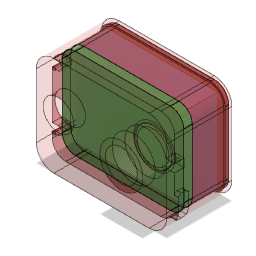
MDCEnclosure (Autodesk Fusion 360 design; units mm, degrees)
Autodesk Fusion 360 part; units mm, degrees
sketch "Board" plane through (0, 0, 0) normal (0, 0, 1) x (1, 0, 0)
  line L0 (4.75, 0) -> (39.105, 0)
  line L1 (43.855, 4.75) -> (43.855, 27.9)
  line L2 (39.105, 32.65) -> (4.75, 32.65)
  line L3 (0, 27.9) -> (0, 4.75)
  arc A0 (4.75, 32.65) -> (0, 27.9) centre (4.75, 27.9) ccw
  arc A1 (43.855, 27.9) -> (39.105, 32.65) centre (39.105, 27.9) ccw
  arc A2 (39.105, 0) -> (43.855, 4.75) centre (39.105, 4.75) ccw
  arc A3 (0, 4.75) -> (4.75, 0) centre (4.75, 4.75) ccw
  line L4 (-0.15, 27.9) -> (-0.15, 4.75)
  arc A4 (-0.15, 4.75) -> (4.75, -0.15) centre (4.75, 4.75) ccw
  line L5 (4.75, -0.15) -> (39.105, -0.15)
  arc A5 (39.105, -0.15) -> (44.005, 4.75) centre (39.105, 4.75) ccw
  line L6 (44.005, 4.75) -> (44.005, 27.9)
  arc A6 (44.005, 27.9) -> (39.105, 32.8) centre (39.105, 27.9) ccw
  line L7 (39.105, 32.8) -> (4.75, 32.8)
  arc A7 (4.75, 32.8) -> (-0.15, 27.9) centre (4.75, 27.9) ccw
  line L8 (-0.35, 27.9) -> (-0.35, 4.75)
  arc A8 (-0.35, 4.75) -> (4.75, -0.35) centre (4.75, 4.75) ccw
  line L9 (4.75, -0.35) -> (39.105, -0.35)
  arc A9 (39.105, -0.35) -> (44.205, 4.75) centre (39.105, 4.75) ccw
  line L10 (44.205, 4.75) -> (44.205, 27.9)
  arc A10 (44.205, 27.9) -> (39.105, 33) centre (39.105, 27.9) ccw
  line L11 (39.105, 33) -> (4.75, 33)
  arc A11 (4.75, 33) -> (-0.35, 27.9) centre (4.75, 27.9) ccw
  line L12 (-0.5, 27.9) -> (-0.5, 4.75)
  arc A12 (-0.5, 4.75) -> (4.75, -0.5) centre (4.75, 4.75) ccw
  line L13 (4.75, -0.5) -> (39.105, -0.5)
  arc A13 (39.105, -0.5) -> (44.355, 4.75) centre (39.105, 4.75) ccw
  line L14 (44.355, 4.75) -> (44.355, 27.9)
  arc A14 (44.355, 27.9) -> (39.105, 33.15) centre (39.105, 27.9) ccw
  line L15 (39.105, 33.15) -> (4.75, 33.15)
  arc A15 (4.75, 33.15) -> (-0.5, 27.9) centre (4.75, 27.9) ccw
  line L16 (21.9275, 32.65) -> (21.9275, 0)
  point P0 (21.9275, 16.325)
  dimension "d329" = 43.855
  dimension "d330" = 32.65
  dimension "d331" = 4.75
  dimension "d332" = 0.15
  dimension "d336" = 0.35
  dimension "d337" = 0.5
  constraint horizontal L0
  constraint vertical L1
  constraint horizontal L2
  constraint vertical L3
  constraint tangent L2 A0
  constraint tangent L3 A0
  constraint tangent L1 A1
  constraint tangent L2 A1
  constraint equal A0 A1
  constraint tangent L0 A2
  constraint tangent L1 A2
  constraint equal A0 A2
  constraint tangent L0 A3
  constraint tangent L3 A3
  constraint equal A0 A3
  constraint midpoint L2 L16.start
  constraint midpoint L0 L16.end
  constraint midpoint L16 P0
  measures "d329" distance of L1 L3
  measures "d330" distance of L0 L2
  measures "d331" radius of A0
ref_plane "WorkPlane7" through (21.9275, 16.325, -3.46) normal (0, 0, 1) x (1, 0, 0)
sketch "MountPoints" plane through (0, 0, -3.46) normal (0, 0, 1) x (1, 0, 0)
  line L0 (-0.15, 29.9) -> (0.44, 29.9)
  line L1 (0.44, 29.9) -> (0.44, 26.9)
  line L2 (0.44, 26.9) -> (-0.15, 26.9)
  line L3 (-0.15, 26.9) -> (-0.15, 29.9)
  line L4 (0.44, 29.9) -> (1.94, 29.9)
  line L5 (3.44, 28.4) -> (3.44, 28.4)
  line L6 (1.94, 26.9) -> (0.44, 26.9)
  line L7 (0.44, 26.9) -> (0.44, 29.9)
  line L8 (0.39, 9.672) -> (1.89, 9.672)
  line L9 (3.39, 8.172) -> (3.39, 8.172)
  line L10 (1.89, 6.672) -> (0.39, 6.672)
  line L11 (0.39, 6.672) -> (0.39, 9.672)
  line L12 (-0.15, 9.672) -> (0.39, 9.672)
  line L13 (0.39, 9.672) -> (0.39, 6.672)
  line L14 (0.39, 6.672) -> (-0.15, 6.672)
  line L15 (-0.15, 6.672) -> (-0.15, 9.672)
  line L16 (-0.15, 27.9) -> (-0.15, 4.75)
  line L17 (44.005, 4.75) -> (44.005, 27.9)
  line L18 (4.75, -0.15) -> (39.105, -0.15)
  line L19 (0.44, 28.4) -> (3.44, 28.4) construction
  line L20 (0.39, 8.172) -> (3.39, 8.172) construction
  line L21 (0, 27.9) -> (0, 4.75) construction
  line L22 (4.75, 0) -> (39.105, 0) construction
  arc A0 (3.44, 28.4) -> (1.94, 29.9) centre (1.94, 28.4) ccw
  arc A1 (1.94, 26.9) -> (3.44, 28.4) centre (1.94, 28.4) ccw
  arc A2 (3.39, 8.172) -> (1.89, 9.672) centre (1.89, 8.172) ccw
  arc A3 (1.89, 6.672) -> (3.39, 8.172) centre (1.89, 8.172) ccw
  line L23 (44.005, 18.892) -> (38.505, 18.892)
  line L24 (38.505, 18.892) -> (38.505, 15.892)
  line L25 (38.505, 15.892) -> (44.005, 15.892)
  line L26 (44.005, 15.892) -> (44.005, 18.892)
  line L27 (44.005, 4.75) -> (44.005, 27.9)
  line L28 (4.75, 0) -> (39.105, 0)
  line L29 (0, 27.9) -> (0, 4.75)
  line L30 (44.005, 17.392) -> (38.505, 17.392)
  point P0 (1.94, 28.4)
  point P1 (1.89, 8.172)
  point P2 (41.9, 17.392)
  dimension "d404" = 3
  dimension "d411" = 3
  dimension "d412" = 1.89
  dimension "d413" = 8.172
  dimension "d418" = 1.94
  dimension "d419" = 28.4
  dimension "d422" = 1.5
  dimension "d572" = 5.5
  dimension "d608" = 17.392
  dimension "d609" = 41.9
  dimension "d610" = 3
  constraint horizontal L0
  constraint vertical L1
  constraint horizontal L2
  constraint vertical L3
  constraint horizontal L4
  constraint horizontal L6
  constraint vertical L7
  constraint horizontal L8
  constraint horizontal L10
  constraint vertical L11
  constraint horizontal L12
  constraint vertical L13
  constraint horizontal L14
  constraint vertical L15
  constraint collinear L1 L7
  constraint collinear L0 L4
  constraint collinear L2 L6
  constraint collinear L3 L16
  constraint collinear L11 L13
  constraint collinear L8 L12
  constraint collinear L10 L14
  constraint collinear L15 L16
  constraint midpoint L1 L19.start
  constraint midpoint L13 L20.start
  constraint midpoint L19 P0
  constraint midpoint L20 P1
  constraint tangent L4 A0
  constraint tangent L6 A1
  constraint equal A0 A1
  constraint tangent L8 A2
  constraint equal A0 A2
  constraint tangent L10 A3
  constraint equal A0 A3
  constraint horizontal L23
  constraint vertical L24
  constraint horizontal L25
  constraint vertical L26
  constraint midpoint L26 L30.start
  constraint midpoint L24 L30.end
  constraint coincident P2 L30
  constraint collinear L26 L27
  measures "d404" distance of L4 L6
  measures "d411" distance of L8 L10
  measures "d412" distance of P1 L21
  measures "d413" distance of P1 L22
  measures "d418" distance of P0 L21
  measures "d419" distance of P0 L22
  measures "d422" radius of A0
  measures "d572" distance of L24 L26
  measures "d608" distance of P2 L28
  measures "d609" distance of P2 L29
  measures "d610" distance of L23 L25
extrude "Front-Sidewalls" add sketch "Board" along normal blind 23.56 thin wall 1.5 on the left open curves L4 A4 L5 A5 L6 A6 L7 A7 makes body 1 in component "Front"
sketch "FrontHoles" plane through (0, 0, 0) normal (0, 0, 1) x (1, 0, 0)
  line L0 (0, 27.9) -> (0, 4.75)
  line L1 (4.75, 0) -> (39.105, 0)
  circle A0 centre (33.5424, 17.392) radius 7.5144
  circle A1 centre (33.5424, 17.392) radius 7.7644
  circle A2 centre (33.5424, 17.392) radius 6.75
  point P0 (6.2926, 17.392)
  point P1 (33.5424, 17.392)
  dimension "d350" = 6.2926
  dimension "d351" = 17.392
  dimension "d352" = 33.5424
  dimension "d353" = 17.392
  dimension "d554" = 15.0287
  dimension "d555" = 15.5287
  dimension "d575" = 13.5
  constraint coincident P1 A0.centre
  measures "d350" distance of P0 L0
  measures "d351" distance of P0 L1
  measures "d352" distance of P1 L0
  measures "d353" distance of P1 L1
  measures "d554" diameter of A0
  measures "d555" diameter of A1
  measures "d575" diameter of A2
extrude "Front-Frontplate" add sketch "Board" along normal blind 4.3 separate body contours L0 L2 L3 A0 A3 L16 | L0 L1 L2 A1 A2 L16 | L4 A4 L5 A5 L6 A6 L7 A7 makes body 2 in component "Front"
hole "Front-MotionSensorHole" at (6.2926, 17.392, 0) direction (0, 0, 1) diameter 11 depth 12 tip angle 118 bodies 2 in component "Front"
extrude "Front-LensProtrusionInside" [suppressed]
extrude "Extrude12" add sketch "FrontHoles" against normal blind 3.46 contours A0 | A2 bodies 2 in component "Front"
extrude "Front-BoardMountPoints" [suppressed]
extrude "Extrude16" add sketch "MountPoints" along normal blind 3.46 contours L0 L1 L2 L3 L7 L16 | L1 L4 L6 L7 A0 A1 | L12 L14 L15 L16 L29 | L11 L12 L13 L14 L29 | L8 L10 L11 L13 A2 A3 | L17 L24 L25 L26 L27 L30 | L17 L23 L24 L26 L27 L30 bodies 2 in component "Front"
extrude "Front-LensProtrusionBoardGap" cut sketch "FrontHoles" along normal blind 0.25 from surface at -3.46 contours A0 | A2 bodies 2 in component "Front"
extrude "Extrude24" [no effect]
extrude "Extrude18" cut sketch "FrontHoles" along normal blind 0.5 from surface at -3.21 contours A2 bodies 2 1 in component "Front"
extrude "Front-LensProtrusionOutside" [suppressed]
extrude "Extrude13" add sketch "FrontHoles" along normal blind 8.74 contours A0 | A1 | A2 bodies 2 in component "Front"
hole "Hole8" at (33.5424, 17.392, -3.46) direction (0, 0, 1) diameter 11.529 depth 20 tip angle 180 bodies 2 in component "Front"
thread "Thread2" "ISO Metric profile 12.0 M12x0.5 6H" major diameter 12.0961 minor diameter 11.5287 pitch 0.5 angle 60 resizes the face on face at (33.8297, 23.1493, 1.1067) from (33.5424, 17.392, -0.71) to (33.5424, 17.392, 8.74) on bodies 2 in component "Front"
hole "Hole10" at (1.94, 28.4, -3.46) at (41.9, 17.392, -3.46) at (1.89, 8.172, -3.46) direction (0, 0, 1) diameter 1.271 depth 5 tip angle 180 bodies 2 1 in component "Front"
thread "Thread4" "ISO Metric profile 1.6 M1.6x0.35 6H" major diameter 1.668 minor diameter 1.271 pitch 0.35 angle 60 resizes the face on face at (41.8683, 18.0267, -0.1267) on face at (1.3283, 28.5721, -1.7933) on face at (1.9217, 8.8067, -1.7933) on bodies 2 in component "Front"
move_body "Align7" bodies 2 to x (1, 0, 0) y (0, 1, 0) z (0, 0, 1) at (0, 0, 19.26) in component "Front"
extrude "Front-BackplateInset" cut sketch "Board" along normal blind 1.5 draft 10 contours L0 L2 L3 A0 A3 L16 | L0 L1 L2 A1 A2 L16 | L4 A4 L5 A5 L6 A6 L7 A7 | L8 A8 L9 A9 L10 A10 L11 A11 | L12 A12 L13 A13 L14 A14 L15 A15 bodies 1 in component "Front"
combine "Front-Combine" operation add target body 1 tool bodies 2 in component "Front"
sketch "USBCPlugCutout" plane through (0, 0, 0) normal (1, 0, 0) x (0, 0, -1) in component "Front"
  line L0 (-22, 4.75) -> (-22, 27.9)
  line L1 (-22, 27.9) -> (-23.5, 27.9)
  line L2 (-23.5, 27.9) -> (-23.5, 4.75)
  line L3 (-23.5, 4.75) -> (-22, 4.75)
  line L4 (-18.715, 19.0109) -> (-17.155, 19.0109)
  line L5 (-16.155, 18.0109) -> (-16.155, 10.6709)
  line L6 (-17.155, 9.6709) -> (-18.715, 9.6709)
  line L7 (-19.715, 10.6709) -> (-19.715, 18.0109)
  arc A0 (-18.715, 19.0109) -> (-19.715, 18.0109) centre (-18.715, 18.0109) ccw
  arc A1 (-16.155, 18.0109) -> (-17.155, 19.0109) centre (-17.155, 18.0109) ccw
  arc A2 (-17.155, 9.6709) -> (-16.155, 10.6709) centre (-17.155, 10.6709) ccw
  arc A3 (-19.715, 10.6709) -> (-18.715, 9.6709) centre (-18.715, 10.6709) ccw
  dimension "d492" = 3.56
  dimension "d493" = 9.34
  dimension "d497" = 1
  dimension "d498" = 1
  dimension "d499" = 1
  constraint horizontal L4
  constraint vertical L5
  constraint vertical L7
  constraint tangent L4 A0
  constraint tangent L7 A0
  constraint tangent L4 A1
  constraint tangent L5 A1
  constraint tangent L5 A2
  constraint tangent L6 A2
  constraint tangent L6 A3
  constraint tangent L7 A3
  constraint equal A2 A3
  measures "d492" distance of L5 L7
  measures "d493" distance of L4 L6
  measures "d497" radius of A0
  measures "d498" radius of A1
  measures "d499" radius of A2
extrude "Extrude9" add sketch "USBCPlugCutout" along normal blind 10 separate body contours L4 L5 L6 L7 A0 A1 A2 A3 makes body 3 in component "Front"
ref_plane "WorkPlane5" through (42.4553, 17.392, 15.7) normal (0, 0, -1) x (-1, 0, 0) in component "Front"
ref_plane "WorkPlane6" through (42.005, 16.325, 11.78) normal (-1, 0, 0) x (0, -1, 0) in component "Front"
move_body "Align3" bodies 3 to x (1, 0, 0) y (0, 1, 0) z (0, 0, 1) at (42.005, 0, 0) in component "Front"
move_body "Align4" bodies 3 to x (1, 0, 0) y (0, 1, 0) z (0, 0, 1) at (0, 0, -0.455) in component "Front"
ref_plane "WorkPlane7" through (21.9275, 0, 0) normal (0, -1, 0) x (1, 0, 0) in component "Front"
ref_plane "WorkPlane9" through (21.9275, 5.2535, 0) normal (0, -1, 0) x (1, 0, 0) in component "Front"
move_body "Align5" bodies 3 to x (1, 0, 0) y (0, 1, 0) z (0, 0, 1) at (0, -9.0874, 0) in component "Front"
combine "Combine3" operation cut target body 1 tool bodies 3 in component "Front"
extrude "Back-Backplate" add sketch "Board" along normal blind 1.5 draft 10 separate body contours L0 L2 L3 A0 A3 L16 | L0 L1 L2 A1 A2 L16 | L4 A4 L5 A5 L6 A6 L7 A7 | L8 A8 L9 A9 L10 A10 L11 A11 makes body 4 in component "Back"
sketch "Sketch1" plane through (0, 0, 0) normal (0, 0, 1) x (1, 0, 0) in component "Battery"
  line L0 (20, 15) -> (-20, 15)
  line L1 (-20, 15) -> (-20, -15)
  line L2 (-20, -15) -> (20, -15)
  line L3 (20, -15) -> (20, 15)
  line L4 (20, 15) -> (-20, -15) construction
  dimension "d443" = 40
  dimension "d444" = 30
  constraint horizontal L0
  constraint vertical L1
  constraint horizontal L2
  constraint vertical L3
  constraint midpoint L4 origin
  measures "d443" distance of L1 L3
  measures "d444" distance of L0 L2
extrude "Extrude1" add sketch "Sketch1" along normal blind 11.2 separate body makes body 5 in component "Battery"
move_body "Align1" bodies 5 to x (1, 0, 0) y (0, 1, 0) z (0, 0, 1) at (21.9275, 16.325, 1.5) in component "Battery"
extrude "Extrude1'" add sketch "Board" along normal blind 3.1 separate body contours L0 L2 L3 A0 A3 L16 | L0 L1 L2 A1 A2 L16 makes body 6 in component "Board"
move_body "Align1'" bodies 6 to x (1, 0, 0) y (0, 1, 0) z (0, 0, 1) at (0, 0, 12.7) in component "Board"
component "Front" placed x (1, 0, 0) y (0, 1, 0) z (0, 0, 1) at (0, 0, 0)
component "Back" placed x (1, 0, 0) y (0, 1, 0) z (0, 0, 1) at (0, 0, 0)
component "Battery" placed x (1, 0, 0) y (0, 1, 0) z (0, 0, 1) at (0, 0, 0)
component "Board" placed x (1, 0, 0) y (0, 1, 0) z (0, 0, 1) at (0, 0, 0)
equation "BoardHeight = 32.65 mm"
equation "BoardWidth = 43.855 mm"
equation "EnclosureThickness = 1.5 mm"
equation "ImageSensorX = 33.5424 mm"
equation "ImageSensorY = 17.392 mm"
equation "MotionSensorX = 6.2926 mm"
equation "MotionSensorY = 17.392 mm"
equation "LensHoleDiameter = 15.1 mm + 0.2 mm + EnclosureMfgTol"
equation "MotionSensorDiameter = 10.4 mm + 0.5 mm + EnclosureMfgTol"
equation "LensProtrusionOutsideThickness = 13.5287 mm + 2 mm"
equation "LensProtrusionDepth = LensThreadDepth - MountPointDepth"
equation "OuterEdgeRadius = 6 mm"
equation "BoardRadius = 4.75 mm"
equation "MountPoint2X = 1.89 mm"
equation "MountPoint2Y = 8.172 mm"
equation "MountPointDepth = USBCReceptacleWidth + 0.3 mm"
equation "MountPoint3X = 41.9 mm"
equation "MountPoint3Y = 17.392 mm"
equation "MountPoint1X = 1.94 mm"
equation "MountPoint1Y = 28.4 mm"
equation "BackplateMountPointDepth = EnclosureDepth - FrontplateThickness"
equation "BackplateMountPointWidth = 1.5 mm"
equation "BackplateMountPointChamfer = BackplateMountPointWidth"
equation "HoleDiameter = 1.3 mm"
equation "BatteryWidth = 40 mm"
equation "BatteryHeight = 30 mm"
equation "BatteryThickness = 11 mm + 0.2 mm"
equation "BackplateOverlap = 0.2 mm"
equation "BackplateHoleOffset = 0.1 mm"
equation "ScrewHeadDiameter = 3 mm"
equation "ScrewHeadHeight = 1 mm"
equation "BackplateThickness = 1.5 mm"
equation "EnclosureDepth = FrontplateThickness + MountPointDepth + BoardThickness + BatteryThickness + BackplateThickness"
equation "BoardThickness = 3.1 mm"
equation "BoardEnclosureGap = 0.15 mm"
equation "USBCReceptacleCutoutWidth = USBCReceptacleWidth + USBCReceptacleTolerance + 2 * EnclosureMfgTol"
equation "USBCReceptacleCutoutHeight = USBCReceptacleHeight + USBCReceptacleTolerance + 2 * EnclosureMfgTol"
equation "USBCReceptacleCutoutRadius = 2.4 mm / 2 - 0.2 mm"
equation "USBCReceptacleY = 5.25348125 mm"
equation "USBCReceptacleWidth = 3.16 mm"
equation "d329 = BoardWidth"
equation "d330 = BoardHeight"
equation "d331 = BoardRadius"
equation "d332 = BoardEnclosureGap"
equation "d333 = EnclosureThickness"
equation "d334 = EnclosureDepth"
equation "d336 = BoardEnclosureGap + BackplateOverlap"
equation "d337 = BoardEnclosureGap + BackplateOverlap + 0.15 mm"
equation "d350 = MotionSensorX"
equation "d351 = MotionSensorY"
equation "d352 = ImageSensorX"
equation "d353 = ImageSensorY"
equation "d354 = FrontplateThickness"
equation "d363 = MotionSensorDiameter"
equation "d372 = EnclosureThickness"
equation "MountPointWidth = 3 mm"
equation "MountPointHeight = 3 mm"
equation "MountPointRadius = 1.5 mm"
equation "d404 = MountPointHeight"
equation "d411 = MountPointHeight"
equation "d412 = MountPoint2X"
equation "d413 = MountPoint2Y"
equation "d418 = MountPoint1X"
equation "d419 = MountPoint1Y"
equation "d422 = MountPointRadius"
equation "d426 = BackplateThickness"
equation "d427 = DovetailAngle"
equation "d443 = BatteryWidth"
equation "d444 = BatteryHeight"
equation "d445 = BatteryThickness"
equation "d479 = BoardThickness"
equation "d492 = USBCReceptacleCutoutWidth"
equation "d493 = USBCReceptacleCutoutHeight"
equation "d497 = USBCReceptacleCutoutRadius"
equation "d498 = USBCReceptacleCutoutRadius"
equation "d499 = USBCReceptacleCutoutRadius"
equation "d502 = EnclosureMfgTol"
equation "d505 = -USBCReceptacleY"
equation "USBCReceptacleHeight = 8.94 mm"
equation "USBCReceptacleTolerance = 0.2 mm"
equation "EnclosureMfgTol = 0.1 mm"
equation "FrontplateThickness = 4.3 mm"
equation "LensThreadDepth = 12.2 mm" comment "Lens threaded region length + lens back focal length (BFL)"
equation "LensProtrusionInsideThickness = 13.0287 mm + 2 mm"
equation "d540 = -MountPointDepth"
equation "d542 = -MountPointDepth"
equation "d544 = LensProtrusionDepth"
equation "d546 = LensProtrusionDepth"
equation "d554 = LensProtrusionInsideThickness"
equation "d555 = LensProtrusionOutsideThickness"
equation "BackplateDovetailAngle = 10 deg"
equation "d575 = LensOringOutsideDiameter"
equation "LensOringOutsideDiameter = 13.5 mm"
equation "LensOringThickness = 1 mm"
equation "LensOringSeatDepth = 0.5 mm"
equation "d590 = MountPointDepth"
equation "d592 = MountPointDepth"
equation "d594 = LensProtrusionBoardGap"
equation "d596 = -MountPointDepth"
equation "LensProtrusionBoardGap = 0.25 mm" comment "Gap between inside lens protrusion and board"
equation "d598 = -MountPointDepth + LensProtrusionBoardGap"
equation "d599 = LensOringSeatDepth"
equation "d601 = -MountPointDepth"
equation "d602 = LensProtrusionBoardGap"
equation "d604 = MountPointHoleDepth"
equation "d608 = MountPoint3Y"
equation "d609 = MountPoint3X"
equation "d610 = MountPointHeight"
equation "d611 = -MountPointDepth"
equation "MountPointHoleDepth = 5 mm"
equation "DovetailAngle = 10 deg"
named bodies: "Body", "Front", "USBCPlugCutout"
